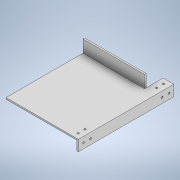
# Autodesk Inventor part: Shooter plate but for an xrail
Saved by Autodesk Inventor 2020.3 (Build 243373010, 373A)
## iProperties
Created: 2020-10-07
Part Number: Shooter plate but for an xrail
Material: Generic
Document SubType Name: Modeling
Designer: Owner
Density: 1 g/cm^3
Appearance: Default
Author: Owner
Autodesk Inventor part; units mm, degrees
ref_plane "YZ Plane" through (0, 0, 0) normal (1, 0, 0) x (0, 1, 0)
ref_plane "XZ Plane" through (0, 0, 0) normal (0, 1, 0) x (-1, 0, 0)
ref_plane "XY Plane" through (0, 0, 0) normal (0, 0, 1) x (1, 0, 0)
sketch "Sketch1" plane through (0, 0, 0) normal (0, 0, 1) x (1, 0, 0)
  line L0 (0, 0) -> (19.05, 0)
  line L1 (19.05, 0) -> (19.05, 19.05)
  line L2 (19.05, 19.05) -> (0, 19.05)
  line L3 (0, 19.05) -> (0, 0)
  line L4 (19.05, 0) -> (22.225, 0)
  line L5 (22.225, 0) -> (22.225, 19.05)
  line L6 (22.225, 19.05) -> (19.05, 19.05)
  line L7 (19.05, 19.05) -> (19.05, 0)
  line L8 (0, 19.05) -> (22.225, 19.05)
  line L9 (22.225, 19.05) -> (22.225, 22.225)
  line L10 (22.225, 22.225) -> (0, 22.225)
  line L11 (0, 22.225) -> (0, 19.05)
  line L12 (0, 19.05) -> (-127, 19.05)
  line L13 (-127, 19.05) -> (-127, 22.225)
  line L14 (-127, 22.225) -> (0, 22.225)
  line L15 (0, 22.225) -> (0, 19.05)
  dimension "d0" = 19.05
  dimension "d1" = 19.05
  dimension "d2" = 3.175
  dimension "d3" = 3.175
  dimension "d4" = 127
  constraints: 32 end point, 8 parallel, 4 horizontal, 4 perpendicular, 2 point on line
  measures "d0" distance of L2.end L1.end
  measures "d1" distance of L1.end L0.end
  measures "d2" distance of L6.end L5.end
  measures "d3" distance of L9.end L8.end
  measures "d4" distance of L13.end L14.end
extrude "Extrusion1" add sketch "Sketch1" along normal blind 196.85 contours L1 L6 L5 L4 | L11 L10 L9 L6 L2 | L12 L13 L14 L11
sketch "Sketch2" plane through (-127, 22.225, 0) normal (0, 1, 0) x (1, 0, 0)
  line L0 (0, 0) -> (127, 0)
  line L1 (127, 0) -> (127, -34.925)
  line L2 (127, -34.925) -> (0, -34.925)
  line L3 (0, -34.925) -> (0, 0)
  dimension "d7" = 34.925
  constraints: 8 end point, 2 parallel, 1 horizontal, 1 perpendicular
  measures "d7" distance of L0.end L1.end
extrude "Extrusion2" cut sketch "Sketch2" against normal blind 25.4
sketch "Sketch3" plane through (-127, 22.225, 196.85) normal (0, 1, 0) x (1, 0, 0)
  line L0 (127, 161.925) -> (0, 161.925) projected
  line L1 (0, 161.925) -> (127, 161.925)
  line L2 (127, 161.925) -> (127, 158.75)
  line L3 (127, 158.75) -> (0, 158.75)
  line L4 (0, 158.75) -> (0, 161.925)
  point P0 (127, 196.85)
  dimension "d10" = 3.175
  constraints: 8 end point, 2 parallel, 1 horizontal, 1 perpendicular
  measures "d10" distance of L1.end L2.end
extrude "Extrusion3" add sketch "Sketch3" along normal blind 25.4
sketch "Sketch4" plane through (-127, 22.225, 196.85) normal (0, 1, 0) x (1, 0, 0)
  line L0 (149.225, 196.85) -> (127, 196.85) projected
  line L1 (149.225, 196.85) -> (149.225, 0) projected
  line L2 (127, 196.85) -> (149.225, 196.85)
  line L3 (149.225, 196.85) -> (149.225, 0)
  line L4 (149.225, 0) -> (127, 0)
  line L5 (127, 0) -> (127, 196.85)
  line L6 (149.225, 0) -> (0, 0) projected
  line L7 (138.1125, 0) -> (138.1125, 196.85)
  line L8 (127, 34.925) -> (149.225, 34.925)
  line L9 (127, 34.925) -> (149.225, 0)
  line L10 (127, 0) -> (149.225, 34.925)
  line L11 (127, 10.3909) -> (149.225, 24.5341)
  line L12 (127, 24.5341) -> (149.225, 10.3909)
  line L13 (127, 196.85) -> (127, 161.925) projected
  line L14 (127, 161.925) -> (149.225, 161.925)
  line L15 (127, 161.925) -> (149.225, 196.85)
  line L16 (149.225, 161.925) -> (127, 196.85)
  line L17 (127, 196.85) -> (127, 172.3159)
  line L18 (149.225, 186.4591) -> (127, 172.3159)
  line L19 (149.225, 172.3159) -> (127, 186.4591)
  line L20 (127, 186.4591) -> (149.225, 186.4591)
  line L21 (127, 10.3909) -> (149.225, 10.3909)
  line L22 (127, 172.3159) -> (149.225, 172.3159)
  line L23 (127, 24.5341) -> (149.225, 24.5341)
  circle A0 centre (138.1125, 10.3909) radius 1.905
  circle A1 centre (138.1125, 24.5341) radius 1.905
  circle A2 centre (138.1125, 172.3159) radius 1.905
  circle A3 centre (138.1125, 186.4591) radius 1.905
  dimension "d13" = 3.81
  dimension "d14" = 3.81
  dimension "d15" = 3.81
  dimension "d16" = 3.81
  constraints: 40 end point, 12 point on line, 11 perpendicular, 5 midpoint, 4 centre point, 3 parallel, 2 horizontal
  measures "d13" diameter of A0
  measures "d14" diameter of A1
  measures "d15" diameter of A2
  measures "d16" diameter of A3
extrude "Extrusion4" cut sketch "Sketch4" against normal blind 25.4 contours A3 L20 L7 | L7 L20 A3 | A3 L7 L20 | L7 A3 L20 | A2 L22 L7 | L7 L22 A2 | A2 L7 L22 | L7 A2 L22 | A1 L23 L7 | L7 L23 A1 | A1 L7 L23 | A0 L21 L7 | L7 L21 A0 | A1 L23 L7 | A0 L7 L21 | L7 A0 L21
sketch "Sketch5" plane through (22.225, 0, 0) normal (1, 0, 0) x (0, 0, -1)
  line L0 (0, 22.225) -> (-196.85, 22.225) projected
  line L1 (0, 0) -> (-196.85, 0) projected
  line L2 (-34.925, 22.225) -> (0, 22.225)
  line L3 (0, 22.225) -> (0, 0)
  line L4 (0, 0) -> (-34.925, 0)
  line L5 (-34.925, 0) -> (-34.925, 22.225)
  line L6 (-196.85, 22.225) -> (-161.925, 22.225)
  line L7 (-161.925, 22.225) -> (-161.925, 0)
  line L8 (-161.925, 0) -> (-196.85, 0)
  line L9 (-196.85, 0) -> (-196.85, 22.225)
  line L10 (-196.85, 19.05) -> (-196.85, 0) projected
  line L11 (-196.85, 11.1125) -> (0, 11.1125)
  line L12 (0, 19.05) -> (0, 0) projected
  line L13 (0, 22.225) -> (-34.925, 0)
  line L14 (-34.925, 22.225) -> (0, 0)
  line L15 (-196.85, 22.225) -> (-161.925, 0)
  line L16 (-161.925, 22.225) -> (-196.85, 0)
  line L17 (-186.4591, 22.225) -> (-172.3159, 0)
  line L18 (-174.2209, 22.225) -> (-170.4109, 22.225) projected
  line L19 (-172.3159, 22.225) -> (-186.4591, 0)
  line L20 (-24.4964, 22.225) -> (-10.3532, 0)
  line L21 (-10.3532, 22.225) -> (-24.4964, 0)
  line L22 (-24.4964, 22.225) -> (-24.4964, 0)
  line L23 (-10.3532, 22.225) -> (-10.3532, 0)
  line L24 (-186.4591, 22.225) -> (-186.4591, 0)
  line L25 (-172.3159, 22.225) -> (-172.3159, 0)
  circle A0 centre (-186.4591, 11.1125) radius 1.905
  circle A1 centre (-172.3159, 11.1125) radius 1.905
  circle A2 centre (-24.4964, 11.1125) radius 1.905
  dimension "d19" = 34.925
  dimension "d20" = 3.81
  dimension "d21" = 3.81
  dimension "d22" = 3.81
  constraints: 42 end point, 12 point on line, 11 parallel, 6 perpendicular, 4 midpoint, 3 centre point, 2 horizontal
  measures "d19" distance of L7.end L8.end
  measures "d20" diameter of A0
  measures "d21" diameter of A1
  measures "d22" diameter of A2
extrude "Extrusion5" cut sketch "Sketch5" against normal blind 25.4 contours A2 L11 L22 | L22 L11 A2 | L11 L22 A2 | A2 L22 L11 | A1 L25 L11 | L11 L25 A1 | L25 L11 A1 | L25 A1 L11 | A0 L24 L11 | L11 L24 A0 | L24 A0 L11 | L11 A0 L24
sketch "Sketch6" plane through (22.225, 0, 0) normal (1, 0, 0) x (0, 0, -1)
  line L0 (0, 22.225) -> (-196.85, 22.225) projected
  line L1 (0, 19.05) -> (0, 0) projected
  line L2 (-34.4902, 22.225) -> (0, 22.225)
  line L3 (0, 22.225) -> (0, 0)
  line L4 (0, 0) -> (-34.4902, 0)
  line L5 (-34.4902, 0) -> (-34.4902, 22.225)
  line L6 (-34.4902, 11.1125) -> (0, 11.1125)
  line L7 (0, 0) -> (0, 22.225) projected
  line L8 (0, 22.225) -> (-34.4902, 0)
  line L9 (-24.4058, 22.225) -> (-10.0843, 0)
  line L10 (0, 0) -> (-196.85, 0) projected
  line L11 (-10.0843, 0) -> (-10.0843, 22.225)
  circle A0 centre (-10.0843, 11.1125) radius 1.905
  dimension "d25" = 3.81
  constraints: 16 end point, 4 point on line, 3 midpoint, 3 perpendicular, 2 parallel, 1 centre point, 1 horizontal
  measures "d25" diameter of A0
extrude "Extrusion6" cut sketch "Sketch6" against normal blind 25.4 contours A0 L6 L11 | L11 L6 A0 | A0 L11 L6 | L6 L11 A0
body "Solid1"
